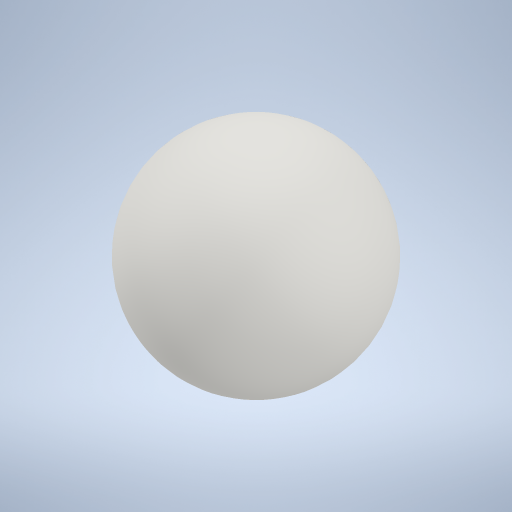
# Autodesk Inventor part: Kugel
Saved by Autodesk Inventor 2024.3 (Build 283343000, 343)
## iProperties
Created: 2025-09-12
Part Number: Kugel
Material: 1.0038 S235JR
Document SubType Name: Modeling
Designer: Dickert.Jonas
Density: 7.86 g/cm^3
Appearance: Stahl
Author: Dickert.Jonas
Autodesk Inventor part; units mm, degrees
ref_plane "YZ Plane" through (0, 0, 0) normal (1, 0, 0) x (0, 1, 0)
ref_plane "XZ Plane" through (0, 0, 0) normal (0, 1, 0) x (-1, 0, 0)
ref_plane "XY Plane" through (0, 0, 0) normal (0, 0, 1) x (1, 0, 0)
sketch "Skizze1" plane through (0, 0, 0) normal (0, 0, 1) x (1, 0, 0)
  arc A0 (0, 3) -> (0, -3) centre (0, 0) ccw
  line L0 (0, -3) -> (0, 3)
  line L1 (0, -4.2) -> (0, 4.2) projected
  constraints: 2 end point, 2 point on circle, 2 point on line, 1 centre point, 1 coincident, 1 vertical
revolve "Umdrehung1" add sketch "Skizze1" angle 360 about axis through (0, -10, 0) along (0, 1, 0)
